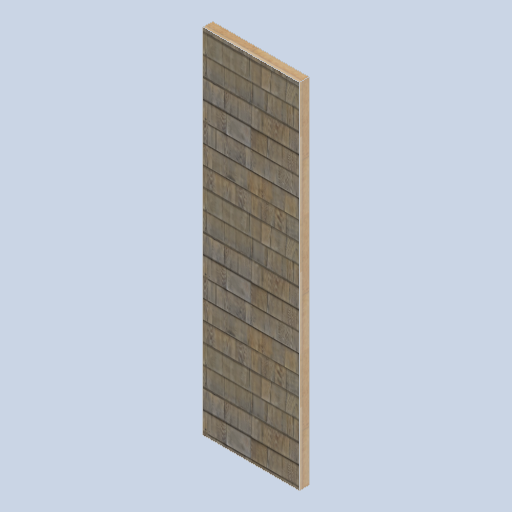
# Autodesk Inventor part: front_wall_block04
Saved by Autodesk Inventor 2024.2 (Build 282272000, 272)
## iProperties
Created: 2024-05-21
Part Number: front_wall_block04
Material: Wood (Maple)
Document SubType Name: Modeling
Designer: LOSTER_1
Density: 0.67 g/cm^3
Appearance: Natural Maple - Glossy Dark Tint
Author: LOSTER_1
Autodesk Inventor part; units mm, degrees
ref_plane "YZ Plane" through (0, 0, 0) normal (1, 0, 0) x (0, 1, 0)
ref_plane "XZ Plane" through (0, 0, 0) normal (0, 1, 0) x (-1, 0, 0)
ref_plane "XY Plane" through (0, 0, 0) normal (0, 0, 1) x (1, 0, 0)
sketch "Sketch1" plane through (0, 0, 0) normal (0, 0, 1) x (1, 0, 0)
  line L0 (-954.2028, 2080.7959) -> (-154.2028, 2082.2883)
  line L1 (-954.2028, -851.5752) -> (-954.2028, 2080.7959)
  line L2 (-154.2028, -851.5752) -> (-954.2028, -851.5752)
  line L3 (-154.2028, 2082.2883) -> (-154.2028, -851.5752)
  point P0 (0, 0)
  point P1 (-163.9907, 369.7807)
  point P2 (-154.2028, 3182.4263)
  constraints: 8 end point, 1 coincident
extrude "Extrusion1" add sketch "Sketch1" along normal blind 80
body "Solid1"
